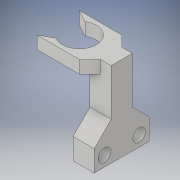
# Autodesk Inventor part: КВ33.044.207 - Крепление вакумной присоски
Saved by Autodesk Inventor 2019 (Build 230136000, 136)
## iProperties
Created: 2019-08-29
Part Number: КВ33.044.207 - Крепление вакумной присоски
Material: Типовые
Document SubType Name: Modeling
Designer: Петров Иван
Density: 1 g/cm^3
Appearance: По умолчанию
Author: Петров Иван
Autodesk Inventor part; units mm, degrees
ref_plane "YZ Plane" through (0, 0, 0) normal (1, 0, 0) x (0, 1, 0)
ref_plane "XZ Plane" through (0, 0, 0) normal (0, 1, 0) x (-1, 0, 0)
ref_plane "XY Plane" through (0, 0, 0) normal (0, 0, 1) x (1, 0, 0)
sketch "Эскиз1" plane through (0, 0, 0) normal (1, 0, 0) x (0, 1, 0)
  line L0 (0, 0) -> (0, -8.197)
  circle A0 centre (0, 0) radius 1.5
  circle A1 centre (0, -8.197) radius 1.5
  line L1 (-2.5, 2.4015) -> (2.5, 2.4015)
  line L2 (2.5, 2.4015) -> (2.5, -10.5985)
  line L3 (2.5, -10.5985) -> (-2.5, -10.5985)
  line L4 (-2.5, -10.5985) -> (-2.5, 2.4015)
  line L5 (-2.5, 2.4015) -> (2.5, -10.5985) construction
  line L6 (2.5, 2.4015) -> (-2.5, -10.5985) construction
  point P0 (0, -4.0985)
  dimension "d0" = 8.197
  dimension "d1" = 3
  dimension "d2" = 3
  dimension "d3" = 5
  dimension "d4" = 13
  constraints: 14 end point, 3 midpoint, 2 centre point, 2 coincident, 2 parallel, 1 horizontal, 1 perpendicular, 1 vertical
  measures "d0" distance of L0.start L0.end
  measures "d1" diameter of A0
  measures "d2" diameter of A1
  measures "d3" distance of L2.end L3.end
  measures "d4" distance of L1.end L2.end
extrude "Выдавливание1" add sketch "Эскиз1" along normal blind 5
sketch "Эскиз2" plane through (0, 2.5, 2.4015) normal (0, 1, 0) x (1, 0, 0)
  line L0 (0, 0) -> (5, 0) projected
  line L1 (2.5, 0) -> (2.5, 13)
  line L2 (0, 13) -> (5, 13) projected
  line L3 (0, 13) -> (0, 0) projected
  line L4 (5, 4) -> (0, 4)
  line L5 (0, 4) -> (0, 9)
  line L6 (0, 9) -> (5, 9)
  line L7 (5, 9) -> (5, 4)
  line L8 (5, 4) -> (0, 9) construction
  line L9 (0, 4) -> (5, 9) construction
  point P0 (0, 2.4015)
  point P1 (2.5, 6.5)
  dimension "d7" = 5
  constraints: 14 end point, 5 midpoint, 2 parallel, 1 horizontal, 1 perpendicular, 1 point on line
  measures "d7" distance of L4.end L5.end
extrude "Выдавливание2" add sketch "Эскиз2" along normal blind 15 contours L3 L6 L1 L4 | L1 L6 L7 L4
sketch "Эскиз3" plane through (0, 0, 0) normal (-1, 0, 0) x (0, 0, 1)
  line L0 (-1.5985, 17.5) -> (-6.5985, 17.5) projected
  line L1 (-4.0985, 17.5) -> (-4.0985, 16)
  line L2 (-9.0985, 14.5) -> (0.9015, 14.5)
  line L3 (0.9015, 14.5) -> (0.9015, 17.5)
  line L4 (0.9015, 17.5) -> (-9.0985, 17.5)
  line L5 (-9.0985, 17.5) -> (-9.0985, 14.5)
  line L6 (-9.0985, 14.5) -> (0.9015, 17.5) construction
  line L7 (0.9015, 14.5) -> (-9.0985, 17.5) construction
  point P0 (0, 0)
  dimension "d10" = 1.5
  dimension "d11" = 10
  dimension "d12" = 3
  constraints: 14 end point, 3 midpoint, 2 parallel, 1 horizontal, 1 perpendicular, 1 vertical
  measures "d10" distance of L1.start L1.end
  measures "d11" distance of L4.end L3.end
  measures "d12" distance of L3.end L2.end
extrude "Выдавливание3" add sketch "Эскиз3" along normal blind 10
sketch "Эскиз4" plane through (0, 17.5, 2.4015) normal (0, 1, 0) x (1, 0, 0)
  line L0 (0, 1.5) -> (-10, 1.5) projected
  line L1 (-5, 1.5) -> (-5, 11.5)
  line L2 (0, 11.5) -> (-10, 11.5) projected
  circle A0 centre (-5, 6.5) radius 4
  line L3 (-7.0808, 9.9162) -> (-10, 11.5)
  line L4 (-10, 1.5) -> (-10, 11.5) projected
  line L5 (-7.0808, 3.0838) -> (-10, 1.5)
  line L6 (-10, 1.5) -> (-10, 11.5)
  point P0 (0, 2.4015)
  dimension "d15" = 8
  constraints: 8 end point, 3 midpoint, 2 point on circle, 1 centre point, 1 collinear, 1 point on line, 1 other
  measures "d15" diameter of A0
extrude "Выдавливание4" cut sketch "Эскиз4" against normal blind 10 contours L4 L3 A0 L5 | A0 L1 | L1 A0
chamfer "Фаска1" distance 2.5 angle 45 2 edges at (0, 16, -1.5985) (0, 16, -6.5985)
chamfer "Фаска2" distance 4 angle 45 2 edges at (2.5, 2.5, -6.5985) (2.5, 2.5, -1.5985)
